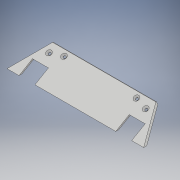
# Autodesk Inventor part: Przod2mm
Saved by Autodesk Inventor 2019 (Build 230136000, 136)
## iProperties
Created: 2022-01-22
Part Number: Przod2mm
Material: Ogólny
Document SubType Name: Modeling
Designer: Michał
Density: 1 g/cm^3
Appearance: Domyślna
Author: Michał
Autodesk Inventor part; units mm, degrees
ref_plane "YZ Plane" through (0, 0, 0) normal (1, 0, 0) x (0, 1, 0)
ref_plane "XZ Plane" through (0, 0, 0) normal (0, 1, 0) x (-1, 0, 0)
ref_plane "XY Plane" through (0, 0, 0) normal (0, 0, 1) x (1, 0, 0)
sketch "Szkic1" plane through (0, 0, 0) normal (1, 0, 0) x (0, 1, 0)
  line L0 (0, 0) -> (22, -38.1051)
  line L1 (22, -38.1051) -> (19.6906, -38.1051)
  line L2 (19.6906, -38.1051) -> (0, -4)
  line L3 (0, -4) -> (0, 0)
  line L4 (22, -38.1051) -> (22, -38.641)
  line L5 (22, -38.641) -> (20, -38.641)
  line L6 (20, -38.641) -> (19.6906, -38.1051)
  dimension "d0" = 2
  dimension "d1" = 22
  dimension "d2" = 30
  dimension "d5" = 2
  constraints: 14 end point, 2 perpendicular, 1 collinear, 1 horizontal, 1 parallel, 1 point on line, 1 vertical
  measures "d0" distance between parallel lines of L2 L0
  measures "d1" distance from line of L3 L0.end
  measures "d2" angle of L3 L2
  measures "d5" distance of L4.end L5.end
extrude "Wyciągnięcie proste1" add sketch "Szkic1" along normal blind 180.175
sketch "Szkic2" plane through (180.175, 22, -38.641) normal (0, 0, -1) x (-1, 0, 0)
  line L0 (180.175, -2) -> (180.175, -22) projected
  line L1 (180.175, 0) -> (0, 0) projected
  line L2 (180.175, -22) -> (180.175, 0)
  line L3 (180.175, 0) -> (158.175, 0)
  line L4 (158.175, 0) -> (180.175, -22)
  line L5 (90.0875, 0) -> (90.0875, -22) construction
  line L6 (180.175, -22) -> (0, -22) construction
  line L7 (0, -2) -> (0, -22)
  line L8 (0, -22) -> (0, 0)
  line L9 (0, 0) -> (22, 0)
  line L10 (22, 0) -> (0, -22)
  line L11 (143.375, -22) -> (164.375, -22)
  line L12 (164.375, -22) -> (164.375, -11.7)
  line L13 (164.375, -11.7) -> (143.375, -11.7)
  line L14 (143.375, -11.7) -> (143.375, -22)
  line L15 (36.8, -22) -> (15.8, -22)
  line L16 (15.8, -22) -> (15.8, -11.7)
  line L17 (15.8, -11.7) -> (36.8, -11.7)
  line L18 (36.8, -11.7) -> (36.8, -22)
  dimension "d6" = 45
  dimension "d9" = 21
  dimension "d10" = 10.3
  dimension "d11" = 15.8
  constraints: 32 end point, 6 symmetric about line, 2 midpoint, 2 parallel, 2 perpendicular, 2 point on line, 1 horizontal
  measures "d6" angle of L0 L4
  measures "d9" distance of L11.end L11.start
  measures "d10" distance of L13.end L11.start
  measures "d11" distance of L0.end L11.end
extrude "Wyciągnięcie proste2" cut sketch "Szkic2" against normal through all
sketch "Szkic3" plane through (22, 22, -38.1051) normal (0, 0.8660254, 0.5) x (1, 0, 0)
  line L0 (-2, -0.5359) -> (138.175, -0.5359) construction
  line L1 (-2, -0.5359) -> (4.3275, -0.5359) construction
  line L2 (4.3275, -0.5359) -> (4.3275, -10.5359) construction
  line L3 (-2, -0.5359) -> (20.3275, -0.5359) construction
  line L4 (20.3275, -0.5359) -> (20.3275, -6.1359) construction
  line L5 (0, 0.4641) -> (136.175, 0.4641) construction
  line L6 (68.0875, 0.4641) -> (68.0875, -44) construction
  line L7 (14.8, -44) -> (121.375, -44) construction
  circle A0 centre (20.3275, -6.1359) radius 1.6
  circle A1 centre (4.3275, -10.5359) radius 1.6
  circle A2 centre (131.8475, -10.5359) radius 1.6
  circle A3 centre (115.8475, -6.1359) radius 1.6
  point P0 (-22, -44)
  dimension "d12" = 6.3275
  dimension "d13" = 10
  dimension "d14" = 22.3275
  dimension "d15" = 5.6
  dimension "d16" = 3.2
  dimension "d17" = 3.2
  constraints: 10 end point, 4 centre point, 2 coincident, 2 midpoint, 2 point on line, 2 vertical, 2 other
  measures "d12" distance of L0.start L1.end
  measures "d13" distance of L1.end L2.end
  measures "d14" distance of L3.end L0.start
  measures "d15" distance of L3.end L4.end
  measures "d16" diameter of A0
  measures "d17" diameter of A1
extrude "Wyciągnięcie proste3" cut sketch "Szkic3" against normal through all
chamfer "Faza1" distance 1.85 distance2 1.75 1 edges at (136.2475, 18.9321, -32.7913) measured on face at (135.7475, 18.9321, -32.7913)
chamfer "Faza2" distance 1.85 distance2 1.75 1 edges at (152.2475, 16.7321, -28.9808) measured on face at (151.7475, 16.7321, -28.9808)
chamfer "Faza3" distance 1.85 distance2 1.75 1 edges at (40.7275, 18.9321, -32.7913) measured on face at (40.2275, 18.9321, -32.7913)
chamfer "Faza4" distance 1.85 distance2 1.75 1 edges at (24.7275, 16.7321, -28.9808) measured on face at (24.2275, 16.7321, -28.9808)
